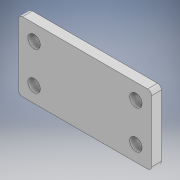
# Autodesk Inventor part: BatteryPlate
Saved by Autodesk Inventor 2020.4 (Build 244396010, 396A)
## iProperties
Created: 2022-09-17
Part Number: BatteryPlate
Material: Generic
Document SubType Name: Sheet Metal
Designer: Val
Density: 1 g/cm^3
Sheet Metal Rule: Default
Appearance: Default
Author: Val
Autodesk Inventor part; units mm, degrees
ref_plane "YZ Plane" through (0, 0, 0) normal (1, 0, 0) x (0, 1, 0)
ref_plane "XZ Plane" through (0, 0, 0) normal (0, 1, 0) x (-1, 0, 0)
ref_plane "XY Plane" through (0, 0, 0) normal (0, 0, 1) x (1, 0, 0)
sketch "Base" plane through (0, 0, 0) normal (0, 0, 1) x (1, 0, 0)
  line L0 (-17.0434, 17.78) -> (17.0434, 17.78)
  line L1 (17.0434, 17.78) -> (17.0434, 0)
  line L2 (17.0434, 0) -> (-17.0434, 0)
  line L3 (-17.0434, 0) -> (-17.0434, 17.78)
  circle A0 centre (13.0434, 13.78) radius 4 construction
  circle A1 centre (-13.0434, 13.78) radius 4 construction
  circle A2 centre (-13.0434, 4) radius 4 construction
  circle A3 centre (13.0434, 4) radius 4 construction
  circle A4 centre (-13.0434, 13.78) radius 1.5875
  circle A5 centre (-13.0434, 4) radius 1.5875
  circle A6 centre (13.0434, 13.78) radius 1.5875
  circle A7 centre (13.0434, 4) radius 1.5875
  point P0 (0, 0)
  point P1 (0, 28.2865)
  point P2 (0, 46.7013)
  point P3 (0, 0)
  dimension "d0" = 17.78
  dimension "d1" = 8
  dimension "d2" = 34.0868
  dimension "d3" = 3.175
  measures "d0" distance of L2.end L0.start
  measures "d1" diameter of A1
  measures "d2" distance of L0.start L0.end
  measures "d3" diameter of A4
extrude "Plate1" add sketch "Base" along normal blind 2.54
fillet "BaseROundFeature" radius 1 4 edges at (-17.0434, 17.78, 1.27) (17.0434, 17.78, 1.27) (-17.0434, 0, 1.27) (17.0434, 0, 1.27)
equation "\"d4\" = Thickness"
equation "\"BendRadius\" = Thickness"
equation "\"BendReliefWidth\" = Thickness"
equation "\"BendReliefDepth\" = 0.5 * Thickness"
equation "\"CornerReliefSize\" = 4 * Thickness"
equation "\"MinimumRemnant\" = 2 * Thickness"
equation "\"TransitionRadius\" = BendRadius"
equation "\"JacobiRadiusSize\" = BendRadius"
equation "\"GapSize\" = Thickness"
equation "\"Thickness\" = 2.54"
body "Solid1"
